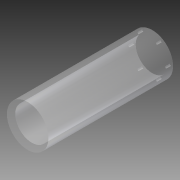
# Autodesk Inventor part: battery_Tube
Saved by Autodesk Inventor 2015 (Build 190159000, 159)
## iProperties
Created: 2011-10-09
Part Number: battery_Tube
Document SubType Name: Modeling
Designer: user
Density: 1 g/cm^3
Material: Generic
Appearance: Polycarbonate - Clear
Author: user
Autodesk Inventor part; units mm, degrees
ref_plane "YZ Plane" through (0, 0, 0) normal (1, 0, 0) x (0, 1, 0)
ref_plane "XZ Plane" through (0, 0, 0) normal (0, 1, 0) x (-1, 0, 0)
ref_plane "XY Plane" through (0, 0, 0) normal (0, 0, 1) x (1, 0, 0)
sketch "Sketch1" plane through (0, 0, 0) normal (0, 0, 1) x (1, 0, 0)
  circle A0 centre (0, 0) radius 35
  circle A1 centre (0, 0) radius 28
  dimension "d0" = 70
  dimension "d1" = 56
  constraints: 2 centre point, 2 coincident
  measures "d0" diameter of A0
  measures "d1" diameter of A1
extrude "Extrusion1" add sketch "Sketch1" along normal blind 210
sketch "Sketch2" plane through (0, 0, 0) normal (0, 0, -1) x (-1, 0, 0)
  circle A0 centre (0, 0) radius 31.5
  constraints: 1 centre point, 1 coincident
extrude "Extrusion2" add sketch "Sketch2" against normal blind 7
sketch "Sketch3" plane through (0, 0, 210) normal (0, 0, 1) x (1, 0, 0)
  circle A0 centre (0, 0) radius 35 projected
  line L0 (35, 0) -> (17.5, -30.3109)
  line L1 (17.5, -30.3109) -> (-17.5, -30.3109)
  line L2 (-17.5, -30.3109) -> (-35, 0)
  line L3 (-35, 0) -> (-17.5, 30.3109)
  line L4 (-17.5, 30.3109) -> (17.5, 30.3109)
  line L5 (17.5, 30.3109) -> (35, 0)
  line L6 (-17.5, 30.3109) -> (17.5, -30.3109)
  line L7 (-17.5, -30.3109) -> (17.5, 30.3109)
  line L8 (-35, 0) -> (35, 0)
  line L9 (-17.5, 30.3109) -> (-15.5, 26.8468)
  line L10 (17.5, 30.3109) -> (15.5, 26.8468)
  line L11 (35, 0) -> (31, 0)
  line L12 (17.5, -30.3109) -> (15.5, -26.8468)
  line L13 (-17.5, -30.3109) -> (-15.5, -26.8468)
  line L14 (-35, 0) -> (-31, 0)
  dimension "d6" = 4
  dimension "d7" = 4
  dimension "d8" = 4
  dimension "d9" = 4
  dimension "d10" = 4
  dimension "d11" = 4
  constraints: 30 end point, 6 point on line, 1 coincident, 1 horizontal, 1 horizontal alignment, 14 other
  measures "d6" distance of L3.end L9.end
  measures "d7" distance of L4.end L10.end
  measures "d8" distance of L0.start L11.end
  measures "d9" distance of L0.end L12.end
  measures "d10" distance of L1.end L13.end
  measures "d11" distance of L2.end L14.end
hole "Hole1" at (-15.5, 26.8468, 210) at (-31, 0, 210) at (-15.5, -26.8468, 210) at (15.5, 26.8468, 210) at (31, 0, 210) at (15.5, -26.8468, 210) direction (0, 0, -1) diameter 3 depth 8 tip angle 118
body "Solid1"
